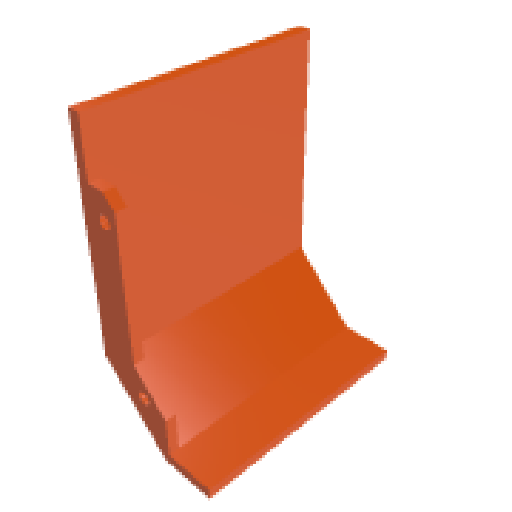
# Autodesk Inventor part: Drag Chain Edge Panel
Saved by Autodesk Inventor 2023.2 (Build 272271000, 271)
## iProperties
Created: 2023-02-24
Part Number: Drag Chain Edge Panel
Material: ABS Plastic
Document SubType Name: Modeling
Designer: remop
Density: 1.06 g/cm^3
Appearance: Smooth - Light Orange
Author: remop
Autodesk Inventor part; units mm, degrees
ref_plane "YZ Plane" through (0, 0, 0) normal (1, 0, 0) x (0, 1, 0)
ref_plane "XZ Plane" through (0, 0, 0) normal (0, 1, 0) x (-1, 0, 0)
ref_plane "XY Plane" through (0, 0, 0) normal (0, 0, 1) x (1, 0, 0)
sketch "Sketch1" plane through (0, 0, 0) normal (0, 0, 1) x (1, 0, 0)
  line L0 (8.7118, -48.8173) -> (8.7118, -78.8173) projected
  line L1 (5.5118, -78.8173) -> (8.7118, -78.8173) projected
  line L2 (5.5118, 131.1827) -> (5.5118, -108.8173) projected
  line L3 (5.5118, 131.1827) -> (5.5118, -141.2563) projected
  line L4 (5.5118, -141.2563) -> (25.5118, -161.2563) projected
  line L5 (25.5118, -161.2563) -> (40.5118, -161.2563) projected
  line L6 (14.7118, -45.3532) -> (8.7118, -48.8173) projected
  line L7 (14.7118, -35.3532) -> (14.7118, -45.3532) projected
  circle A0 centre (11.7118, -40.3532) radius 1.85 projected
  line L8 (8.7118, -31.8891) -> (14.7118, -35.3532) projected
  line L9 (8.7118, -78.8173) -> (8.7118, -140.2136)
  line L10 (8.7118, -140.2136) -> (26.7544, -158.2563)
  line L11 (26.7544, -158.2563) -> (40.5118, -158.2563)
  line L12 (40.5118, -158.2563) -> (40.5118, -161.2563)
  point P0 (0, 0)
  point P1 (33.0118, -161.2563)
  dimension "d0" = 3
  dimension "d1" = 3
  constraints: 8 end point, 2 perpendicular, 1 midpoint, 1 parallel, 1 vertical
  measures "d0" distance between parallel lines of L4 L10
  measures "d1" distance from line of point (33.012, -161.256) L11
extrude "Extrusion1" add sketch "Sketch1" along normal blind 64 contours L1 L9 L10 L11 L12 L5 L4 L3 L2
sketch "Sketch2" plane through (0, 0, 64) normal (0, 0, 1) x (1, 0, 0)
  line L0 (8.7118, -140.2136) -> (8.7118, -78.8173) projected
  line L1 (26.7544, -158.2563) -> (8.7118, -140.2136) projected
  circle A0 centre (12.7118, -101.131) radius 1.75
  circle A1 centre (19.3686, -145.2136) radius 1.75
  line L2 (26.7544, -158.2563) -> (26.7544, -146.9426)
  line L3 (26.7544, -146.9426) -> (16.7118, -136.8999)
  line L4 (16.7118, -136.8999) -> (16.7118, -97.131)
  line L5 (16.7118, -97.131) -> (13.3981, -93.8173)
  line L6 (13.3981, -93.8173) -> (8.7118, -93.8173)
  line L7 (8.7118, -140.2136) -> (8.7118, -78.8173) projected
  point P0 (0, 0)
  dimension "d4" = 4
  dimension "d5" = 4
  dimension "d6" = 3.5
  dimension "d7" = 4
  dimension "d8" = 4
  dimension "d9" = 45
  dimension "d10" = 4
  dimension "d11" = 5
  dimension "d12" = 15
  constraints: 10 end point, 2 centre point, 2 parallel, 1 equal length, 1 equal radius, 1 perpendicular, 1 point on line, 1 vertical
  measures "d4" distance from line of L1 A1.centre
  measures "d5" distance from line of L0 A0.centre
  measures "d6" diameter of A1
  measures "d7" distance from line of A0.centre L4
  measures "d8" horizontal distance of A0.centre L4.end
  measures "d9" angle of L5 L4
  measures "d10" distance from line of L3 A1.centre
  measures "d11" vertical distance of L0.start A1.centre
  measures "d12" distance from line of L0.end L6
extrude "Extrusion2" add sketch "Sketch2" against normal blind 3
equation "\"d1\" = d0"
equation "\"d5\" = d4"
equation "\"d7\" = d5"
equation "\"d8\" = d7"
equation "\"d10\" = d4"
body "Solid1"
